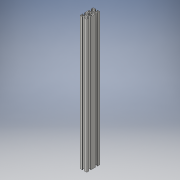
# Autodesk Inventor part: 20 in double rail
Saved by Autodesk Inventor 2016 SP2 (Build 200236200, 236)
## iProperties
Created: 2018-01-27
Part Number: 20 in double rail
Material: Generic
Document SubType Name: Modeling
Designer: CAD
Density: 1 g/cm^3
Appearance: Default
Author: CAD
Autodesk Inventor part; units mm, degrees
ref_plane "YZ Plane" through (0, 0, 0) normal (1, 0, 0) x (0, 1, 0)
ref_plane "XZ Plane" through (0, 0, 0) normal (0, 1, 0) x (-1, 0, 0)
ref_plane "XY Plane" through (0, 0, 0) normal (0, 0, 1) x (1, 0, 0)
sketch "Sketch1" plane through (0, 0, 0) normal (0, 1, 0) x (-1, 0, 0)
  circle A0 centre (0, 0) radius 2.54
  line L0 (-4.5085, 4.5085) -> (4.5085, 4.5085)
  line L1 (-4.5085, -4.5085) -> (4.5085, -4.5085)
  line L2 (4.5085, 4.5085) -> (4.5085, -4.5085)
  line L3 (-4.5085, 4.5085) -> (-4.5085, -4.5085)
  line L4 (-3.0896, 4.5085) -> (-11.2811, 12.7)
  line L5 (-4.5085, 3.0537) -> (-12.7, 11.2452)
  line L6 (12.7, 12.7) -> (-12.7, 12.7)
  line L7 (-12.7, 12.7) -> (-12.7, 4.0005)
  line L8 (-10.668, 4.0005) -> (-10.668, 9.2132)
  line L9 (-9.2491, 10.668) -> (-3.3655, 10.668)
  line L10 (-12.7, 12.7) -> (-3.3655, 12.7)
  line L11 (-2.7305, 11.303) -> (-2.7305, 12.065)
  line L12 (-12.065, 3.3655) -> (-11.303, 3.3655)
  arc A1 (-12.7, 4.0005) -> (-12.065, 3.3655) centre (-12.065, 4.0005) ccw
  arc A2 (-11.303, 3.3655) -> (-10.668, 4.0005) centre (-11.303, 4.0005) ccw
  arc A3 (-3.3655, 10.668) -> (-2.7305, 11.303) centre (-3.3655, 11.303) ccw
  arc A4 (-2.7305, 12.065) -> (-3.3655, 12.7) centre (-3.3655, 12.065) ccw
  arc A5 (-3.3655, -11.303) -> (-4.0005, -10.668) centre (-4.0005, -11.303) ccw
  line L13 (-3.3655, -12.065) -> (-3.3655, -11.303)
  arc A6 (-4.0005, -12.7) -> (-3.3655, -12.065) centre (-4.0005, -12.065) ccw
  line L14 (-3.0537, -4.5085) -> (-11.2452, -12.7)
  line L15 (-10.668, -9.2491) -> (-10.668, -3.3655)
  line L16 (-4.5085, -3.0896) -> (-12.7, -11.2811)
  line L17 (-12.7, -12.7) -> (-12.7, -3.3655)
  arc A7 (-10.668, -3.3655) -> (-11.303, -2.7305) centre (-11.303, -3.3655) ccw
  line L18 (-11.303, -2.7305) -> (-12.065, -2.7305)
  arc A8 (-12.065, -2.7305) -> (-12.7, -3.3655) centre (-12.065, -3.3655) ccw
  line L19 (-4.0005, -10.668) -> (-9.2132, -10.668)
  line L20 (-12.7, -12.7) -> (-4.0005, -12.7)
  arc A9 (11.303, -3.3655) -> (10.668, -4.0005) centre (11.303, -4.0005) ccw
  line L21 (12.065, -3.3655) -> (11.303, -3.3655)
  arc A10 (12.7, -4.0005) -> (12.065, -3.3655) centre (12.065, -4.0005) ccw
  line L22 (4.5085, -3.0537) -> (12.7, -11.2452)
  line L23 (9.2491, -10.668) -> (3.3655, -10.668)
  line L24 (3.0896, -4.5085) -> (11.2811, -12.7)
  line L25 (12.7, -12.7) -> (3.3655, -12.7)
  arc A11 (3.3655, -10.668) -> (2.7305, -11.303) centre (3.3655, -11.303) ccw
  line L26 (2.7305, -11.303) -> (2.7305, -12.065)
  arc A12 (2.7305, -12.065) -> (3.3655, -12.7) centre (3.3655, -12.065) ccw
  line L27 (10.668, -4.0005) -> (10.668, -9.2132)
  line L28 (12.7, -12.7) -> (12.7, -4.0005)
  arc A13 (3.3655, 11.303) -> (4.0005, 10.668) centre (4.0005, 11.303) ccw
  line L29 (3.3655, 12.065) -> (3.3655, 11.303)
  arc A14 (4.0005, 12.7) -> (3.3655, 12.065) centre (4.0005, 12.065) ccw
  line L30 (3.0537, 4.5085) -> (11.2452, 12.7)
  line L31 (10.668, 9.2491) -> (10.668, 3.3655)
  line L32 (4.5085, 3.0896) -> (12.7, 11.2811)
  line L33 (12.7, 12.7) -> (12.7, 3.3655)
  arc A15 (10.668, 3.3655) -> (11.303, 2.7305) centre (11.303, 3.3655) ccw
  line L34 (11.303, 2.7305) -> (12.065, 2.7305)
  arc A16 (12.065, 2.7305) -> (12.7, 3.3655) centre (12.065, 3.3655) ccw
  line L35 (4.0005, 10.668) -> (9.2132, 10.668)
  line L36 (12.7, 12.7) -> (4.0005, 12.7)
  line L37 (-4.5085, 3.0537) -> (-4.5085, 4.5085)
  line L38 (-3.0896, 4.5085) -> (-4.5085, 4.5085)
  line L39 (-12.7, -12.7) -> (-4.0005, -12.7)
  line L40 (-4.0005, -10.668) -> (-9.2132, -10.668)
  line L41 (-10.668, -9.2491) -> (-10.668, -3.3655)
  line L42 (-12.7, -12.7) -> (-12.7, -3.3655)
  line L43 (-11.303, -2.7305) -> (-12.065, -2.7305)
  arc A17 (-10.668, -3.3655) -> (-11.303, -2.7305) centre (-11.303, -3.3655) ccw
  arc A18 (-12.065, -2.7305) -> (-12.7, -3.3655) centre (-12.065, -3.3655) ccw
  line L44 (-4.5085, -3.0896) -> (-4.5085, -4.5085)
  line L45 (-4.5085, -3.0896) -> (-12.7, -11.2811)
  line L46 (-3.0537, -4.5085) -> (-4.5085, -4.5085)
  line L47 (-3.0537, -4.5085) -> (-11.2452, -12.7)
  line L48 (-4.5085, -4.5085) -> (-4.5085, 4.5085)
  circle A19 centre (0, 0) radius 2.54
  line L49 (-4.5085, -4.5085) -> (4.5085, -4.5085)
  line L50 (-3.3655, -12.065) -> (-3.3655, -11.303)
  arc A20 (-4.0005, -12.7) -> (-3.3655, -12.065) centre (-4.0005, -12.065) ccw
  arc A21 (-3.3655, -11.303) -> (-4.0005, -10.668) centre (-4.0005, -11.303) ccw
  line L51 (12.7, -12.7) -> (12.7, -4.0005)
  line L52 (10.668, -4.0005) -> (10.668, -9.2132)
  line L53 (9.2491, -10.668) -> (3.3655, -10.668)
  line L54 (12.7, -12.7) -> (3.3655, -12.7)
  line L55 (2.7305, -11.303) -> (2.7305, -12.065)
  arc A22 (3.3655, -10.668) -> (2.7305, -11.303) centre (3.3655, -11.303) ccw
  arc A23 (2.7305, -12.065) -> (3.3655, -12.7) centre (3.3655, -12.065) ccw
  line L56 (3.0896, -4.5085) -> (4.5085, -4.5085)
  line L57 (3.0896, -4.5085) -> (11.2811, -12.7)
  line L58 (4.5085, -3.0537) -> (4.5085, -4.5085)
  line L59 (4.5085, -3.0537) -> (12.7, -11.2452)
  line L60 (4.5085, -4.5085) -> (-4.5085, -4.5085)
  circle A24 centre (0, 0) radius 2.54
  line L61 (4.5085, -4.5085) -> (4.5085, 4.5085)
  line L62 (12.065, -3.3655) -> (11.303, -3.3655)
  arc A25 (12.7, -4.0005) -> (12.065, -3.3655) centre (12.065, -4.0005) ccw
  arc A26 (11.303, -3.3655) -> (10.668, -4.0005) centre (11.303, -4.0005) ccw
  line L63 (12.7, 12.7) -> (4.0005, 12.7)
  line L64 (4.0005, 10.668) -> (9.2132, 10.668)
  line L65 (10.668, 9.2491) -> (10.668, 3.3655)
  line L66 (12.7, 12.7) -> (12.7, 3.3655)
  line L67 (11.303, 2.7305) -> (12.065, 2.7305)
  arc A27 (10.668, 3.3655) -> (11.303, 2.7305) centre (11.303, 3.3655) ccw
  arc A28 (12.065, 2.7305) -> (12.7, 3.3655) centre (12.065, 3.3655) ccw
  line L68 (4.5085, 3.0896) -> (4.5085, 4.5085)
  line L69 (4.5085, 3.0896) -> (12.7, 11.2811)
  line L70 (3.0537, 4.5085) -> (4.5085, 4.5085)
  line L71 (3.0537, 4.5085) -> (11.2452, 12.7)
  line L72 (4.5085, 4.5085) -> (4.5085, -4.5085)
  circle A29 centre (0, 0) radius 2.54
  line L73 (4.5085, 4.5085) -> (-4.5085, 4.5085)
  line L74 (3.3655, 12.065) -> (3.3655, 11.303)
  arc A30 (4.0005, 12.7) -> (3.3655, 12.065) centre (4.0005, 12.065) ccw
  arc A31 (3.3655, 11.303) -> (4.0005, 10.668) centre (4.0005, 11.303) ccw
  line L75 (4.0005, -14.732) -> (9.2132, -14.732)
  line L76 (4.0005, -14.732) -> (9.2132, -14.732)
  arc A32 (3.3655, -14.097) -> (4.0005, -14.732) centre (4.0005, -14.097) ccw
  arc A33 (3.3655, -14.097) -> (4.0005, -14.732) centre (4.0005, -14.097) ccw
  line L77 (3.3655, -13.335) -> (3.3655, -14.097)
  line L78 (3.3655, -13.335) -> (3.3655, -14.097)
  line L79 (10.668, -16.1509) -> (10.668, -22.0345)
  line L80 (10.668, -16.1509) -> (10.668, -22.0345)
  line L81 (3.0537, -20.8915) -> (11.2452, -12.7)
  line L82 (3.0537, -20.8915) -> (11.2452, -12.7)
  line L83 (4.5085, -22.3104) -> (12.7, -14.1189)
  line L84 (4.5085, -22.3104) -> (12.7, -14.1189)
  line L85 (12.7, -12.7) -> (12.7, -22.0345)
  line L86 (12.7, -12.7) -> (12.7, -22.0345)
  line L87 (12.7, -12.7) -> (4.0005, -12.7)
  line L88 (12.7, -12.7) -> (4.0005, -12.7)
  circle A34 centre (0, -25.4) radius 2.54
  circle A35 centre (0, -25.4) radius 2.54
  circle A36 centre (0, -25.4) radius 2.54
  circle A37 centre (0, -25.4) radius 2.54
  line L89 (4.5085, -20.8915) -> (-4.5085, -20.8915)
  line L90 (-4.5085, -20.8915) -> (4.5085, -20.8915)
  line L91 (-4.5085, -20.8915) -> (-4.5085, -29.9085)
  line L92 (-4.5085, -29.9085) -> (-4.5085, -20.8915)
  line L93 (3.0537, -20.8915) -> (4.5085, -20.8915)
  line L94 (4.5085, -29.9085) -> (4.5085, -20.8915)
  line L95 (4.5085, -20.8915) -> (4.5085, -29.9085)
  line L96 (4.5085, -20.8915) -> (4.5085, -29.9085)
  line L97 (-4.5085, -28.4896) -> (-4.5085, -29.9085)
  line L98 (-3.0537, -29.9085) -> (-4.5085, -29.9085)
  line L99 (-4.5085, -29.9085) -> (4.5085, -29.9085)
  line L100 (4.5085, -29.9085) -> (-4.5085, -29.9085)
  line L101 (-4.5085, -29.9085) -> (4.5085, -29.9085)
  line L102 (4.5085, -22.3104) -> (4.5085, -20.8915)
  line L103 (-4.5085, -22.3463) -> (-4.5085, -20.8915)
  arc A38 (-4.0005, -38.1) -> (-3.3655, -37.465) centre (-4.0005, -37.465) ccw
  arc A39 (-4.0005, -38.1) -> (-3.3655, -37.465) centre (-4.0005, -37.465) ccw
  line L104 (-10.668, -34.6491) -> (-10.668, -28.7655)
  line L105 (-10.668, -34.6491) -> (-10.668, -28.7655)
  line L106 (-3.3655, -37.465) -> (-3.3655, -36.703)
  line L107 (-3.3655, -37.465) -> (-3.3655, -36.703)
  arc A40 (-3.3655, -36.703) -> (-4.0005, -36.068) centre (-4.0005, -36.703) ccw
  arc A41 (-3.3655, -36.703) -> (-4.0005, -36.068) centre (-4.0005, -36.703) ccw
  line L108 (-12.7, -38.1) -> (-4.0005, -38.1)
  line L109 (-12.7, -38.1) -> (-4.0005, -38.1)
  line L110 (-3.0537, -29.9085) -> (-11.2452, -38.1)
  line L111 (-3.0537, -29.9085) -> (-11.2452, -38.1)
  line L112 (-4.5085, -28.4896) -> (-12.7, -36.6811)
  line L113 (-4.5085, -28.4896) -> (-12.7, -36.6811)
  line L114 (-12.7, -38.1) -> (-12.7, -28.7655)
  line L115 (-12.7, -38.1) -> (-12.7, -28.7655)
  line L116 (-4.0005, -36.068) -> (-9.2132, -36.068)
  line L117 (-4.0005, -36.068) -> (-9.2132, -36.068)
  line L118 (12.065, -28.7655) -> (11.303, -28.7655)
  line L119 (12.065, -28.7655) -> (11.303, -28.7655)
  arc A42 (11.303, -28.7655) -> (10.668, -29.4005) centre (11.303, -29.4005) ccw
  arc A43 (11.303, -28.7655) -> (10.668, -29.4005) centre (11.303, -29.4005) ccw
  line L120 (10.668, -29.4005) -> (10.668, -34.6132)
  line L121 (10.668, -29.4005) -> (10.668, -34.6132)
  line L122 (12.7, -38.1) -> (12.7, -29.4005)
  line L123 (12.7, -38.1) -> (12.7, -29.4005)
  line L124 (4.5085, -28.4537) -> (12.7, -36.6452)
  line L125 (4.5085, -28.4537) -> (12.7, -36.6452)
  line L126 (3.0896, -29.9085) -> (11.2811, -38.1)
  line L127 (3.0896, -29.9085) -> (11.2811, -38.1)
  line L128 (12.7, -38.1) -> (3.3655, -38.1)
  line L129 (12.7, -38.1) -> (3.3655, -38.1)
  line L130 (9.2491, -36.068) -> (3.3655, -36.068)
  line L131 (9.2491, -36.068) -> (3.3655, -36.068)
  arc A44 (12.7, -29.4005) -> (12.065, -28.7655) centre (12.065, -29.4005) ccw
  arc A45 (12.7, -29.4005) -> (12.065, -28.7655) centre (12.065, -29.4005) ccw
  line L132 (4.5085, -28.4537) -> (4.5085, -29.9085)
  line L133 (3.0896, -29.9085) -> (4.5085, -29.9085)
  arc A46 (10.668, -22.0345) -> (11.303, -22.6695) centre (11.303, -22.0345) ccw
  arc A47 (10.668, -22.0345) -> (11.303, -22.6695) centre (11.303, -22.0345) ccw
  line L134 (11.303, -22.6695) -> (12.065, -22.6695)
  line L135 (11.303, -22.6695) -> (12.065, -22.6695)
  arc A48 (12.065, -22.6695) -> (12.7, -22.0345) centre (12.065, -22.0345) ccw
  arc A49 (12.065, -22.6695) -> (12.7, -22.0345) centre (12.065, -22.0345) ccw
  line L136 (-2.7305, -14.097) -> (-2.7305, -13.335)
  arc A50 (-3.3655, -14.732) -> (-2.7305, -14.097) centre (-3.3655, -14.097) ccw
  arc A51 (-2.7305, -13.335) -> (-3.3655, -12.7) centre (-3.3655, -13.335) ccw
  arc A52 (4.0005, -12.7) -> (3.3655, -13.335) centre (4.0005, -13.335) ccw
  arc A53 (4.0005, -12.7) -> (3.3655, -13.335) centre (4.0005, -13.335) ccw
  line L137 (-3.0896, -20.8915) -> (-11.2811, -12.7)
  line L138 (-12.7, -12.7) -> (-12.7, -21.3995)
  line L139 (-10.668, -21.3995) -> (-10.668, -16.1868)
  line L140 (-9.2491, -14.732) -> (-3.3655, -14.732)
  line L141 (-12.7, -12.7) -> (-3.3655, -12.7)
  line L142 (-3.0896, -20.8915) -> (-4.5085, -20.8915)
  line L143 (-12.065, -22.0345) -> (-11.303, -22.0345)
  arc A54 (-12.7, -21.3995) -> (-12.065, -22.0345) centre (-12.065, -21.3995) ccw
  arc A55 (-11.303, -22.0345) -> (-10.668, -21.3995) centre (-11.303, -21.3995) ccw
  arc A56 (-10.668, -28.7655) -> (-11.303, -28.1305) centre (-11.303, -28.7655) ccw
  line L144 (-11.303, -28.1305) -> (-12.065, -28.1305)
  arc A57 (-12.065, -28.1305) -> (-12.7, -28.7655) centre (-12.065, -28.7655) ccw
  arc A58 (-10.668, -28.7655) -> (-11.303, -28.1305) centre (-11.303, -28.7655) ccw
  arc A59 (-12.065, -28.1305) -> (-12.7, -28.7655) centre (-12.065, -28.7655) ccw
  line L145 (-11.303, -28.1305) -> (-12.065, -28.1305)
  arc A60 (3.3655, -36.068) -> (2.7305, -36.703) centre (3.3655, -36.703) ccw
  line L146 (2.7305, -36.703) -> (2.7305, -37.465)
  arc A61 (2.7305, -37.465) -> (3.3655, -38.1) centre (3.3655, -37.465) ccw
  arc A62 (2.7305, -37.465) -> (3.3655, -38.1) centre (3.3655, -37.465) ccw
  line L147 (2.7305, -36.703) -> (2.7305, -37.465)
  arc A63 (3.3655, -36.068) -> (2.7305, -36.703) centre (3.3655, -36.703) ccw
  line L148 (-4.5085, -22.3463) -> (-12.7, -14.1548)
  point P0 (-12.7, 3.3655)
  point P1 (-2.7305, 12.7)
  point P2 (-3.3655, -12.7)
  point P3 (-12.7, -2.7305)
  point P4 (12.7, -3.3655)
  point P5 (2.7305, -12.7)
  point P6 (3.3655, 12.7)
  point P7 (12.7, 2.7305)
  point P8 (-3.3655, -12.7)
  point P9 (-12.7, -2.7305)
  point P10 (12.7, -3.3655)
  point P11 (2.7305, -12.7)
  point P12 (3.3655, 12.7)
  point P13 (12.7, 2.7305)
  point P14 (3.3655, -12.7)
  point P15 (3.3655, -12.7)
  point P16 (12.7, -22.6695)
  point P17 (12.7, -22.6695)
  point P18 (-3.3655, -38.1)
  point P19 (-3.3655, -38.1)
  point P20 (-12.7, -28.1305)
  point P21 (-12.7, -28.1305)
  point P22 (12.7, -28.7655)
  point P23 (12.7, -28.7655)
  point P24 (2.7305, -38.1)
  point P25 (2.7305, -38.1)
  point P26 (-2.7305, -12.7)
  point P27 (-12.7, -22.0345)
  dimension "d12" = 5.08
  dimension "d13" = 9.017
  dimension "d14" = 4.5085
  dimension "d15" = 4.5085
  dimension "d16" = 4.5085
  dimension "d17" = 2.032
  dimension "d18" = 1.0033
  dimension "d19" = 135
  dimension "d20" = 9.3345
  dimension "d21" = 2.032
  dimension "d22" = 2.032
  dimension "d23" = 0.635
  dimension "d24" = 9.3345
  dimension "d25" = 360
  dimension "d26" = 360
  dimension "d28" = 16.0655
  dimension "d29" = 0
  dimension "d30" = 25.4
  dimension "d36" = 5.08
  dimension "d37" = 9.017
  dimension "d38" = 4.5085
  dimension "d41" = 2.032
  dimension "d42" = 1.0033
  dimension "d44" = 9.3345
  dimension "d45" = 2.032
  dimension "d47" = 0.635
  dimension "d49" = 360
  dimension "d50" = 360
  dimension "d53" = 25.4
  dimension "d54" = 15.4305
  constraints: 298 end point, 116 point on line, 112 point on circle, 64 centre point, 17 tangent, 8 horizontal, 8 vertical, 6 coincident, 6 equal radius, 2 collinear, 2 parallel, 2 perpendicular, 600 other
  measures "d12" diameter of A0
  measures "d13" distance between parallel lines of L0 L1
  measures "d14" distance from line of L0 point (0, 0)
  measures "d15" distance from line of point (0, 0) L2
  measures "d16" distance from line of point (0, 0) L3
  measures "d17" distance between parallel lines of L5 L4
  measures "d18" distance from line of L0.start L4
  measures "d19" angle of L0 L4
  measures "d20" distance of L7.start point (-12.7, 3.365)
  measures "d21" distance between parallel lines of L7 L8
  measures "d22" distance between parallel lines of L6 L9
  measures "d23" radius of A1
  measures "d24" distance of L7.start L10.end
  measures "d28" distance between parallel lines of L62 L6
  measures "d29" distance from line of L6.start L66
  measures "d30" distance from line of point (-12.7, -12.7) L66
  measures "d36" diameter of A34
  measures "d37" distance between parallel lines of L90 L99
  measures "d38" distance from line of L90 point (0, -25.4)
  measures "d41" distance between parallel lines of L148 L137
  measures "d42" distance from line of L90.start L137
  measures "d44" distance of L141.start point (-12.7, -22.034)
  measures "d45" distance between parallel lines of L138 L139
  measures "d47" radius of A54
  measures "d53" distance from line of point (-12.7, -38.1) L86
  measures "d54" distance from line of point (-12.7, -38.1) L135
extrude "Extrusion1" add sketch "Sketch1" along normal blind 508 contours L3 L5 L7 L6 L4 L0 | L0 L2 L1 L3 | L30 L6 L33 L32 L2 L0 | L4 L6 A4 L11 A3 L9 | L3 L1 L14 L20 L17 L16 | L8 A2 L12 A1 L7 L5 | L35 A13 L29 A14 L6 L30 | L16 L17 A8 L18 A7 L15 | L22 L28 L25 L24 L1 L2 | L32 L33 A16 L34 A15 L31 | L19 A5 L13 A6 L20 L14 | L20 L137 L89 L91 L148 L138 | L27 A9 L21 A10 L28 L22 | L24 L25 A12 L26 A11 L23 | L20 L141 A51 L136 A50 L140 L137 | L148 L139 A55 L143 A54 L138 | L25 L85 L83 L94 L89 L81 | L81 L75 A32 L77 A52 L25 | L89 L94 L99 L98 L91 | L85 A48 L134 A46 L79 L83 | L91 L98 L110 L108 L114 L112 | L112 L114 A57 L144 A56 L104 | L124 L122 L128 L126 L99 L94 | L116 A40 L106 A38 L108 L110 | L120 A42 L118 A44 L122 L124 | L126 L128 A61 L146 A60 L130
equation "\"d24\" = d20"
body "Solid1"
